Autodesk Inventor part; units mm, degrees
(part 2 of 2)
sketch "Sketch3" plane through (0, 3.048, 0) normal (0, 1, 0) x (1, 0, 0)
  spline S0 degree 2 poles (-81.5448, 214.057) (-85.0967, 212.1778) (-85.0967, 211.6202) knots 0 0 0 1 1 1 projected
  spline S1 degree 2 poles (-85.0967, 211.6202) (-85.0967, 211.0213) (-84.6217, 210.6909) knots 0 0 0 1 1 1 projected
  spline S2 degree 2 poles (-84.6217, 210.6909) (-83.9403, 210.1747) (-81.1112, 208.8324) knots 0 0 0 1 1 1 projected
  spline S3 degree 2 poles (-74.09, 206.9945) (-68.9894, 209.1009) (-66.4494, 210.8974) knots 0 0 0 1 1 1 projected
  spline S4 degree 2 poles (-66.4494, 210.8974) (-66.2429, 211.0213) (-66.2429, 211.3311) knots 0 0 0 1 1 1 projected
  spline S5 degree 2 poles (-66.2429, 211.3311) (-66.2429, 212.0952) (-66.532, 212.343) knots 0 0 0 1 1 1 projected
  line L0 (-62.9388, 385.7031) -> (-62.9388, 371.062) projected
  line L1 (-62.9388, 371.062) -> (-88.3388, 371.062) projected
  line L2 (-88.3388, 371.062) -> (-88.3388, 385.827) projected
  line L3 (-85.0967, 385.6205) -> (-85.0967, 374.2835) projected
  line L4 (-85.0967, 374.2835) -> (-77.2908, 374.2835) projected
  line L5 (-77.2908, 374.2835) -> (-77.2908, 379.5906) projected
  line L6 (-74.09, 379.5906) -> (-74.09, 374.2835) projected
  line L7 (-74.09, 374.2835) -> (-66.2429, 374.2835) projected
  line L8 (-66.2429, 374.2835) -> (-66.2429, 385.7031) projected
  line L9 (-88.3388, 331.7643) -> (-88.3388, 337.0301) projected
  line L10 (-85.138, 338.3104) -> (-85.138, 332.5696) projected
  line L11 (-77.1463, 326.4158) -> (-67.4406, 326.4158) projected
  line L12 (-67.2341, 336.0802) -> (-71.199, 336.0802) projected
  line L13 (-71.199, 336.0802) -> (-71.199, 332.5696) projected
  line L14 (-74.5443, 332.6935) -> (-74.5443, 339.3843) projected
  line L15 (-74.5443, 339.3843) -> (-67.1308, 339.3843) projected
  line L16 (-66.9243, 323.1943) -> (-77.8277, 323.1943) projected
  line L17 (-68.4731, 310.9074) -> (-68.4731, 303.8449) projected
  line L18 (-88.3801, 307.4381) -> (-88.2975, 307.5207) projected
  line L19 (-62.9388, 237.7017) -> (-62.9388, 227.4591) projected
  line L20 (-62.9388, 227.4591) -> (-88.3388, 227.4591) projected
  line L21 (-88.3388, 227.4591) -> (-88.3388, 238.0734) projected
  spline S6 degree 2 poles (-64.0952, 214.6558) (-62.9388, 213.5407) (-62.9388, 211.6202) knots 0 0 0 1 1 1 projected
  spline S7 degree 2 poles (-62.9388, 211.6202) (-62.9388, 209.6997) (-64.2191, 208.502) knots 0 0 0 1 1 1 projected
  line L22 (-75.5768, 203.5252) -> (-76.4648, 203.5252) projected
  spline S8 degree 2 poles (-87.265, 208.7911) (-88.2562, 209.7823) (-88.3388, 211.5789) knots 0 0 0 1 1 1 projected
  line L23 (-88.3388, 211.5789) -> (-88.3388, 211.9713) projected
  spline S9 degree 2 poles (-88.3388, 211.9713) (-88.4214, 213.8917) (-86.3357, 215.2547) knots 0 0 0 1 1 1 projected
  line L24 (-76.7746, 188.9874) -> (-64.5289, 195.9052) projected
  line L25 (-76.8572, 185.0225) -> (-76.8572, 182.7922) projected
  line L26 (-76.8572, 182.7922) -> (-64.1365, 182.7922) projected
  line L27 (-64.3843, 179.5914) -> (-88.3388, 179.5914) projected
  line L28 (-88.3388, 179.5914) -> (-88.3388, 191.5893) projected
  line L29 (-123.4102, 399.1569) -> (-100.4056, 399.1569) projected
  spline S10 degree 2 poles (-100.4056, 399.1569) (-99.2079, 399.1569) (-99.2079, 396.7201) knots 0 0 0 1 1 1 projected
  spline S11 degree 2 poles (-99.2079, 396.7201) (-99.2079, 394.3247) (-100.8806, 394.3247) knots 0 0 0 1 1 1 projected
  spline S12 degree 2 poles (-100.8806, 394.3247) (-102.1196, 394.3247) (-102.2848, 394.6757) knots 0 0 0 1 1 1 projected
  spline S13 degree 2 poles (-102.2848, 394.6757) (-102.4294, 395.3159) (-102.6359, 395.9148) knots 0 0 0 1 1 1 projected
  line L30 (-102.6359, 395.9148) -> (-113.1263, 395.9148) projected
  line L31 (-113.1263, 395.9148) -> (-113.1263, 384.2679) projected
  spline S14 degree 2 poles (-113.1263, 384.2679) (-113.1263, 383.9788) (-114.0762, 383.0289) (-114.324, 383.0289) knots 0 0 0 0.5 1 1 1 projected
  line L32 (-114.324, 383.0289) -> (-123.3689, 383.0289) projected
  spline S15 degree 2 poles (-123.3689, 383.0289) (-123.7406, 383.0289) (-124.6079, 384.144) (-124.6079, 384.4744) knots 0 0 0 0.5 1 1 1 projected
  line L33 (-124.6079, 384.4744) -> (-124.6079, 397.67) projected
  spline S16 degree 2 poles (-124.6079, 397.67) (-124.6079, 398.0417) (-123.7612, 399.1569) (-123.4102, 399.1569) knots 0 0 0 0.5 1 1 1 projected
  line L34 (-110.896, 351.3512) -> (-101.9957, 351.3512) projected
  line L35 (-99.2079, 348.5221) -> (-99.2079, 340.1793) projected
  line L36 (-102.512, 340.1793) -> (-102.512, 348.0471) projected
  line L37 (-102.512, 348.0471) -> (-110.2972, 348.0471) projected
  line L38 (-110.2972, 348.0471) -> (-110.2972, 338.3827) projected
  line L39 (-110.2972, 338.3827) -> (-124.6079, 338.3827) projected
  line L40 (-124.6079, 338.3827) -> (-124.6079, 349.9056) projected
  line L41 (-121.3658, 350.1534) -> (-121.3658, 341.6248) projected
  line L42 (-121.3658, 341.6248) -> (-113.5599, 341.6248) projected
  line L43 (-113.5599, 341.6248) -> (-113.5599, 348.7699) projected
  line L44 (-124.6079, 279.6736) -> (-100.7154, 279.6736) projected
  line L45 (-100.7567, 276.3695) -> (-119.9203, 276.3695) projected
  line L46 (-115.563, 273.21) -> (-115.2739, 273.21) projected
  line L47 (-117.9172, 268.2746) -> (-120.1474, 266.5813) projected
  line L48 (-120.1474, 266.5813) -> (-100.6534, 266.5813) projected
  line L49 (-100.6534, 263.3598) -> (-124.6079, 263.3598) projected
  line L50 (-124.6079, 263.3598) -> (-124.6079, 267.5931) projected
  line L51 (-124.6079, 267.5931) -> (-118.991, 271.4548) projected
  line L52 (-118.991, 271.4548) -> (-124.6079, 275.5642) projected
  line L53 (-124.6079, 275.5642) -> (-124.6079, 279.6736) projected
  line L54 (-104.7422, 251.0728) -> (-104.7422, 244.0104) projected
  line L55 (-124.6492, 247.6035) -> (-124.5666, 247.6861) projected
  line L56 (-124.6079, 207.8722) -> (-120.1681, 207.8722) projected
  line L57 (-120.4985, 204.7126) -> (-121.1799, 204.7126) projected
  line L58 (-121.3038, 201.326) -> (-100.5295, 201.326) projected
  line L59 (-100.7567, 197.9806) -> (-121.3451, 197.9806) projected
  line L60 (-121.3451, 197.9806) -> (-121.3451, 194.8624) projected
  line L61 (-119.8583, 191.5583) -> (-124.6079, 191.5583) projected
  line L62 (-124.6079, 191.5583) -> (-124.6079, 207.8722) projected
  line L63 (-99.2079, 230.1333) -> (-99.2079, 215.4922) projected
  line L64 (-99.2079, 215.4922) -> (-124.6079, 215.4922) projected
  line L65 (-124.6079, 215.4922) -> (-124.6079, 230.2572) projected
  line L66 (-121.3658, 230.0507) -> (-121.3658, 218.7136) projected
  line L67 (-121.3658, 218.7136) -> (-113.5599, 218.7136) projected
  line L68 (-113.5599, 218.7136) -> (-113.5599, 224.0208) projected
  line L69 (-110.3591, 224.0208) -> (-110.3591, 218.7136) projected
  line L70 (-110.3591, 218.7136) -> (-102.512, 218.7136) projected
  line L71 (-102.512, 218.7136) -> (-102.512, 230.1333) projected
  line L72 (-107.4268, 324.9187) -> (-100.4056, 324.9187) projected
  line L73 (-100.4469, 321.6972) -> (-107.4268, 321.6972) projected
  line L74 (-107.4268, 321.6972) -> (-107.4268, 312.0328) projected
  line L75 (-107.4268, 312.0328) -> (-123.3689, 312.0328) projected
  line L76 (-123.4102, 315.2336) -> (-110.8134, 315.2336) projected
  line L77 (-110.8134, 315.2336) -> (-110.8134, 321.6972) projected
  line L78 (-110.8134, 321.6972) -> (-120.6224, 321.6972) projected
  line L79 (-120.5398, 324.9187) -> (-110.8134, 324.9187) projected
  line L80 (-124.6079, 375.4089) -> (-114.6338, 375.4089) projected
  line L81 (-108.3354, 368.8627) -> (-100.5295, 368.8627) projected
  line L82 (-100.7567, 365.5174) -> (-109.1407, 365.5174) projected
  line L83 (-115.4598, 372.1048) -> (-121.3658, 372.1048) projected
  line L84 (-121.3658, 372.1048) -> (-121.3658, 362.3991) projected
  line L85 (-124.6079, 360.5406) -> (-124.6079, 375.4089) projected
  spline S17 degree 2 poles (-64.0952, 262.5235) (-62.9388, 261.4083) (-62.9388, 259.4878) knots 0 0 0 1 1 1 projected
  spline S18 degree 2 poles (-62.9388, 259.4878) (-62.9388, 257.5674) (-64.2191, 256.3696) knots 0 0 0 1 1 1 projected
  line L86 (-75.5768, 251.3929) -> (-76.4648, 251.3929) projected
  spline S19 degree 2 poles (-87.265, 256.6587) (-88.2562, 257.65) (-88.3388, 259.4465) knots 0 0 0 1 1 1 projected
  line L87 (-88.3388, 259.4465) -> (-88.3388, 259.8389) projected
  spline S20 degree 2 poles (-88.3388, 259.8389) (-88.4214, 261.7594) (-86.3357, 263.1223) knots 0 0 0 1 1 1 projected
  line L88 (-62.9388, 289.9678) -> (-62.9388, 275.3267) projected
  line L89 (-62.9388, 275.3267) -> (-88.3388, 275.3267) projected
  line L90 (-88.3388, 275.3267) -> (-88.3388, 290.0917) projected
  line L91 (-85.0967, 289.8852) -> (-85.0967, 278.5482) projected
  line L92 (-85.0967, 278.5482) -> (-77.2908, 278.5482) projected
  line L93 (-77.2908, 278.5482) -> (-77.2908, 283.8553) projected
  line L94 (-74.09, 283.8553) -> (-74.09, 278.5482) projected
  line L95 (-74.09, 278.5482) -> (-66.2429, 278.5482) projected
  line L96 (-66.2429, 278.5482) -> (-66.2429, 289.9678) projected
  line L97 (-62.9388, 362.0171) -> (-62.9388, 347.1282) projected
  line L98 (-62.9388, 347.1282) -> (-87.0998, 347.1282) projected
  line L99 (-87.1411, 350.329) -> (-66.2429, 350.329) projected
  line L100 (-66.2429, 350.329) -> (-66.2429, 361.7693) projected
  line L101 (-62.9388, 408.274) -> (-62.9388, 398.7542) projected
  line L102 (-66.2429, 398.9813) -> (-66.2429, 407.7991) projected
  line L103 (-66.4081, 407.8817) -> (-66.5939, 407.8817) projected
  line L104 (-88.3388, 398.1966) -> (-88.3388, 407.448) projected
  line L105 (-84.9934, 406.8904) -> (-84.9934, 398.2792) projected
  circle A0 centre (-11.9063, 413.5437) radius 5.5563 projected
  circle A1 centre (-11.9063, 186.5312) radius 5.5562 projected
  circle A2 centre (-135.7313, 11.9062) radius 5.5562 projected
  circle A3 centre (-189.7062, 545.3062) radius 5.5563 projected
  line L106 (0, 590.55) -> (0, 0) projected
  line L107 (-203.2, 590.55) -> (0, 590.55) projected
  line L108 (-203.2, 514.35) -> (-203.2, 590.55) projected
  line L109 (-165.1, 514.35) -> (-203.2, 514.35) projected
  line L110 (-165.1, 47.625) -> (-165.1, 514.35) projected
  line L111 (-203.2, 47.625) -> (-165.1, 47.625) projected
  line L112 (-203.2, 0) -> (-203.2, 47.625) projected
  line L113 (0, 0) -> (-203.2, 0) projected
  line L114 (-85.0967, 190.9904) -> (-85.0967, 182.7922) projected
  line L115 (-85.0967, 182.7922) -> (-80.0993, 182.7922) projected
  line L116 (-80.0993, 182.7922) -> (-80.0993, 190.9904) projected
  line L117 (-73.9455, 237.8256) -> (-73.9455, 230.6805) projected
  line L118 (-73.9455, 230.6805) -> (-66.2842, 230.6805) projected
  line L119 (-66.2842, 230.6805) -> (-66.2842, 237.7017) projected
  line L120 (-69.3611, 240.3449) -> (-70.9099, 240.3449) projected
  line L121 (-85.0967, 237.5984) -> (-85.0967, 230.6805) projected
  line L122 (-85.0967, 230.6805) -> (-77.4147, 230.6805) projected
  line L123 (-77.4147, 230.6805) -> (-77.4147, 237.5984) projected
  line L124 (-108.0463, 250.2468) -> (-118.516, 247.6448) projected
  line L125 (-118.516, 247.6448) -> (-108.0463, 244.9809) projected
  line L126 (-108.0463, 244.9809) -> (-108.0463, 250.2468) projected
  line L127 (-108.0463, 250.2468) -> (-118.516, 247.6448) projected
  spline S21 degree 2 poles (-81.5448, 261.9246) (-85.0967, 260.0454) (-85.0967, 259.4878) knots 0 0 0 1 1 1 projected
  spline S22 degree 2 poles (-85.0967, 259.4878) (-85.0967, 258.889) (-84.6217, 258.5586) knots 0 0 0 1 1 1 projected
  spline S23 degree 2 poles (-84.6217, 258.5586) (-83.9403, 258.0423) (-81.1112, 256.7) knots 0 0 0 1 1 1 projected
  spline S24 degree 2 poles (-74.09, 254.8622) (-68.9894, 256.9685) (-66.4494, 258.7651) knots 0 0 0 1 1 1 projected
  spline S25 degree 2 poles (-66.4494, 258.7651) (-66.2429, 258.889) (-66.2429, 259.1987) knots 0 0 0 1 1 1 projected
  spline S26 degree 2 poles (-66.2429, 259.1987) (-66.2429, 259.9628) (-66.532, 260.2106) knots 0 0 0 1 1 1 projected
  spline S27 degree 2 poles (-66.532, 260.2106) (-66.9656, 260.5617) (-70.1045, 262.1311) knots 0 0 0 1 1 1 projected
  line L128 (-82.2469, 307.4794) -> (-71.7772, 304.8155) projected
  line L129 (-71.7772, 304.8155) -> (-71.7772, 310.0813) projected
  line L130 (-71.7772, 310.0813) -> (-82.2469, 307.4794) projected
  line L131 (-121.3658, 395.9148) -> (-121.3658, 386.2504) projected
  line L132 (-121.3658, 386.2504) -> (-116.3684, 386.2504) projected
  line L133 (-116.3684, 386.2504) -> (-116.3684, 395.9148) projected
  line L134 (-116.3684, 395.9148) -> (-121.3658, 395.9148) projected
  line L135 (-108.0463, 244.9809) -> (-108.0463, 250.2468) projected
  line L136 (-108.0463, 244.9809) -> (-104.7422, 244.0104)
  line L137 (-108.0463, 250.2468) -> (-104.7422, 251.0728)
  line L138 (-85.0967, 182.7922) -> (-80.0993, 182.7922) projected
  line L139 (-76.8572, 182.7922) -> (-64.1365, 182.7922) projected
  line L140 (-80.0993, 182.7922) -> (-76.8572, 182.7922)
  line L141 (-73.9455, 230.6805) -> (-73.9455, 227.4591)
  line L142 (-88.3388, 227.4591) -> (-62.9388, 227.4591) projected
  line L143 (-66.2842, 230.6805) -> (-66.2842, 227.4591)
  line L144 (-62.9388, 227.4591) -> (-88.3388, 227.4591) projected
  line L145 (-77.4147, 230.6805) -> (-77.4147, 237.5984) projected
  line L146 (-77.4147, 230.6805) -> (-77.4147, 227.4591)
  line L147 (-85.0967, 230.6805) -> (-85.0967, 227.4591)
  line L148 (-116.3684, 395.9148) -> (-116.3684, 399.1569)
  line L149 (-121.3658, 395.9148) -> (-121.3658, 399.1569)
  line L150 (-123.4102, 399.1569) -> (-100.4056, 399.1569) projected
  line L151 (-71.7772, 304.8155) -> (-68.4731, 303.8449)
  line L152 (-71.7772, 310.0813) -> (-68.4731, 310.9074)
  line L153 (-68.5616, 209.5905) -> (-63.3922, 209.5905)
  line L154 (-68.4049, 213.4005) -> (-63.2518, 213.4005)
  spline S28 degree 2 poles (-66.532, 212.343) (-66.9656, 212.694) (-70.1045, 214.2635) knots 0 0 0 1 1 1 projected
  line L155 (-87.8512, 209.5905) -> (-82.6693, 209.5905)
  line L156 (-88.0662, 213.4005) -> (-82.7487, 213.4005)
  line L157 (-87.9464, 257.6535) -> (-83.0537, 257.6535)
  line L158 (-87.9692, 261.4635) -> (-82.399, 261.4635)
  line L159 (-68.232, 257.6432) -> (-63.3037, 257.6432)
  line L160 (-68.7839, 261.4635) -> (-63.3366, 261.4635)
  line L161 (-80.0993, 182.7922) -> (-80.0993, 190.9904) projected
  line L162 (-80.0993, 185.8402) -> (-75.4997, 185.8402)
  spline S29 degree 2 poles (-67.9981, 190.2883) (-73.5118, 187.0462) (-76.8572, 185.0225) knots 0 0 0 1 1 1 projected
  point P0 (-80.0993, 185.0225)
  dimension "d32" = 3.81
  dimension "d33" = 3.81
  dimension "d34" = 3.81
  dimension "d35" = 3.8203
  dimension "d51" = 3.048
  constraints: 40 end point, 8 horizontal, 8 point on line, 7 perpendicular, 1 collinear, 1 vertical, 229 other
  measures "d32" distance between parallel lines of L154 L153
  measures "d33" distance between parallel lines of L156 L155
  measures "d34" distance between parallel lines of L157 L158
  measures "d35" distance between parallel lines of L160 L159
  measures "d51" distance between parallel lines of L140 L162
extrude "Extrusion4" add sketch "Sketch3" against normal up to surface (3.048 mm away) contours S0 S1 S2 L155 S8 L23 S9 L156 | S3 S4 S5 S28 L154 S6 S7 L153 | L17 L151 L129 L152 | L20 L141 L118 L143 | L20 L147 L122 L146 | L25 L140 L116 L162 S29 | L29 L148 L134 L149 | L54 L136 L126 L137 | S17 S18 L159 S24 S25 S26 S27 L160 | S19 L87 S20 L158 S21 S22 S23 L157
sketch "Sketch4" plane through (0, 0, 0) normal (0, -1, 0) x (1, 0, 0)
  line L0 (0, -590.55) -> (-203.2, -590.55) projected
  line L1 (-128.2154, -527.05) -> (-128.2154, -590.55)
  line L2 (-165.1, -514.35) -> (-165.1, -47.625) projected
  line L3 (-150.8125, -498.8028) -> (-165.1, -498.8028)
  line L4 (-100.0125, -527.05) -> (-144.4625, -527.05)
  line L5 (-150.8125, -520.7) -> (-150.8125, -476.25)
  line L6 (-144.4625, -469.9) -> (-100.0125, -469.9)
  line L7 (-93.6625, -476.25) -> (-93.6625, -520.7)
  arc A0 (-150.8125, -520.7) -> (-144.4625, -527.05) centre (-144.4625, -520.7) ccw
  arc A1 (-144.4625, -469.9) -> (-150.8125, -476.25) centre (-144.4625, -476.25) ccw
  arc A2 (-93.6625, -476.25) -> (-100.0125, -469.9) centre (-100.0125, -476.25) ccw
  arc A3 (-100.0125, -527.05) -> (-93.6625, -520.7) centre (-100.0125, -520.7) ccw
  line L8 (-203.2, 0) -> (0, 0) projected
  line L9 (0, -590.55) -> (0, 0) projected
  line L10 (0, -176.2125) -> (-50.8, -176.2125)
  line L11 (0, 0) -> (0, -590.55) projected
  circle A4 centre (-50.8, -149.225) radius 26.9875
  line L12 (0, -176.2125) -> (0, -122.2375)
  line L13 (0, -122.2375) -> (-50.8, -122.2375)
  point P0 (-150.8125, -469.9)
  point P1 (-150.8125, -527.05)
  point P2 (-93.6625, -469.9)
  dimension "d38" = 63.5
  dimension "d39" = 14.2875
  dimension "d40" = 57.15
  dimension "d41" = 57.15
  dimension "d42" = 6.35
  dimension "d45" = 176.2125
  dimension "d47" = 50.8
  constraints: 18 end point, 12 point on line, 10 point on circle, 10 tangent, 5 centre point, 4 perpendicular, 3 equal radius, 3 horizontal, 2 parallel, 1 collinear
  measures "d38" distance of L1.start L1.end
  measures "d39" distance of L3.start L3.end
  measures "d40" distance of point (-150.812, -469.9) point (-93.663, -469.9)
  measures "d41" distance of point (-150.812, -527.05) point (-150.812, -469.9)
  measures "d42" radius of A0
  measures "d45" distance between parallel lines of L8 L10
  measures "d47" distance from line of L9 A4.centre
extrude "Extrusion5" cut sketch "Sketch4" against normal up to surface (3.048 mm away)
ref_plane "Work Plane2" through (0, 0, -295.275) normal (0, 0, -1) x (-1, 0, 0)
fillet "Fillet1" radius 5.08 10 edges at (-203.2, 1.524, -590.55) (-203.2, 1.524, -514.35) (-165.1, 1.524, -514.35) (-203.2, 1.524, -47.625) (-165.1, 1.524, -47.625) (-203.2, 1.524, 0) (0, 1.524, 0) (0, 1.524, -122.2375) (0, 1.524, -176.2125) (0, 1.524, -590.55)
sketch "Sketch5" plane through (0, 0, 0) normal (0, -1, 0) x (1, 0, 0)
  line L0 (-5.08, -590.55) -> (-198.12, -590.55) projected
  line L1 (-203.2, -585.47) -> (-203.2, -519.43) projected
  line L2 (-198.12, 0) -> (-5.08, 0) projected
  line L3 (-203.2, -42.545) -> (-203.2, -5.08) projected
  line L4 (-189.7062, -590.55) -> (-189.7062, -571.5)
  circle A0 centre (-189.7062, -545.3062) radius 5.5563 projected
  line L5 (-195.2625, -545.3062) -> (-195.2625, -590.55)
  circle A1 centre (-189.7062, -565.9438) radius 5.5563
  circle A2 centre (-135.7313, -11.9062) radius 5.5562 projected
  line L6 (-135.7313, 0) -> (-135.7313, -26.9875)
  line L7 (-141.2875, 0) -> (-141.2875, -45.1845)
  circle A3 centre (-135.7313, -32.5437) radius 5.5562
  point P0 (0, 0)
  dimension "d56" = 11.1125
  dimension "d52" = 19.05
  dimension "d53" = 26.9875
  constraints: 8 end point, 8 vertical, 4 point on line, 2 vertical alignment, 1 horizontal alignment, 1 perpendicular, 1 tangent, 5 other
  measures "d52" distance of L4.start L4.end
  measures "d53" distance of L6.start L6.end
extrude "Extrusion6" cut sketch "Sketch5" against normal up to next contours A1 | A3
sketch "Sketch6" plane through (0, 0, 0) normal (0, -1, 0) x (1, 0, 0)
  circle A0 centre (-135.7313, -11.9062) radius 5.5562 projected
  circle A1 centre (-189.7062, -545.3062) radius 5.5563 projected
  point P0 (0, 0)
extrude "Extrusion7" add sketch "Sketch6" against normal up to surface (3.048 mm away)
equation "\"BendRadius\" = Thickness"
equation "\"BendReliefWidth\" = Thickness"
equation "\"BendReliefDepth\" = 0.5 * Thickness"
equation "\"CornerReliefSize\" = 4 * Thickness"
equation "\"MinimumRemnant\" = 2 * Thickness"
equation "\"TransitionRadius\" = BendRadius"
equation "\"JacobiRadiusSize\" = BendRadius"
equation "\"GapSize\" = Thickness"
equation "\"d20\" = BendRadius"
equation "\"Thickness\" = 3.048"
body "Solid1"
